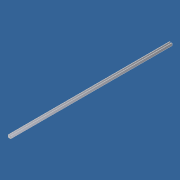
# Autodesk Inventor part: GE-11041-02
Saved by Autodesk Inventor 2012 (Build 160160000, 160)
## iProperties
Created: 2010-09-30
Part Number: GE-11041-02
Document SubType Name: Modeling
Designer: mcyr
Density: 1 g/cm^3
Description: Glass Holder
Material: Default
Title: Glass Holder
Author: mcyr
Autodesk Inventor part; units mm, degrees
ref_plane "YZ Plane" through (0, 0, 0) normal (1, 0, 0) x (0, 1, 0)
ref_plane "XZ Plane" through (0, 0, 0) normal (0, 1, 0) x (-1, 0, 0)
ref_plane "XY Plane" through (0, 0, 0) normal (0, 0, 1) x (1, 0, 0)
sketch "Sketch1" plane through (0, 0, 0) normal (0, 0, 1) x (1, 0, 0)
  line L0 (-19.1418, 21.9502) -> (-22.3168, 21.9502)
  line L1 (-22.3168, 21.9502) -> (-22.3168, 2.9002)
  line L2 (-22.3168, 2.9002) -> (-3.2668, 2.9002)
  line L3 (-3.2668, 2.9002) -> (-3.2668, 21.9502)
  line L4 (-3.2668, 21.9502) -> (-6.4418, 21.9502)
  line L5 (-6.4418, 21.9502) -> (-6.4418, 6.0752)
  line L6 (-6.4418, 6.0752) -> (-19.1418, 6.0752)
  line L7 (-19.1418, 6.0752) -> (-19.1418, 21.9502)
  point P0 (0, 0)
  dimension "d0" = 12.7
  dimension "d2" = 3.175
  dimension "d3" = 3.175
  dimension "d4" = 19.05
  dimension "d5" = 15.875
  dimension "d6" = 15.875
  constraints: 16 end point, 5 parallel, 1 collinear, 1 horizontal, 1 perpendicular
  measures "d0" distance of L5.end L6.end
  measures "d2" distance of L0.start L0.end
  measures "d3" distance of L3.end L4.end
  measures "d4" distance of L0.end L1.end
  measures "d5" distance of L4.end L5.end
  measures "d6" distance from line of L6.end L0
extrude "Extrusion1" add sketch "Sketch1" along normal blind 1238.25
body "Solid1"
